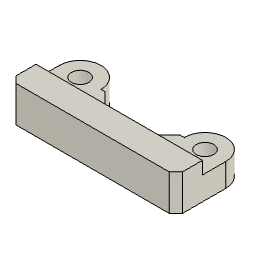
ADXL Nozzle Mount v8 (Autodesk Fusion 360 design; units mm, degrees)
Autodesk Fusion 360 part; units mm, degrees
note: some values were not read from the file. Set by a fixed rule: which sketch regions a step uses.
sketch "Sketch1" plane through (0, 0, 0) normal (0, 0, 1) x (1, 0, 0)
  circle A0 centre (-10.1925, 0) radius 2.5
  circle A1 centre (-25.1925, 0) radius 2.5
  circle A2 centre (-25.1925, 0) radius 1.6
  circle A3 centre (-10.1925, 0) radius 1.6
  line L0 (-27.6925, 0) -> (-7.6925, 0)
  line L1 (-7.6925, 0) -> (-7.6925, -6)
  line L2 (-7.6925, -6) -> (-27.6925, -6)
  line L3 (-27.6925, -6) -> (-27.6925, 0)
  line L4 (-27.6925, 0) -> (-22.6925, 0)
  line L5 (-20.6925, 0) -> (-14.6925, 0)
  line L6 (-14.6925, 0) -> (-14.6925, -2.5)
  line L7 (-14.6925, -2.5) -> (-20.6925, -2.5)
  line L8 (-20.6925, -2.5) -> (-20.6925, 0)
  line L9 (-27.6925, 0) -> (-2.5588, 0)
  line L10 (-7.6925, -2.8) -> (-27.6925, -2.8)
  line L11 (-27.6925, -2.8) -> (-27.6925, 0)
  circle A4 centre (-25.1925, 0) radius 1.05
  circle A5 centre (-10.1925, 0) radius 1.05
  dimension "d1" = 5
  dimension "d3" = 5
  dimension "d4" = 15
  dimension "d6" = 3.2
  dimension "d7" = 3.2
  dimension "d10" = 6
  dimension "d11" = 5
  dimension "d13" = 2.5
  dimension "d14" = 2.8
  dimension "d21" = 6
  dimension "d22" = 2.1
  dimension "d23" = 2.1
  constraint concentric A1 A2
  constraint concentric A0 A3
  constraint horizontal L0
  constraint coincident A1 L0.start
  constraint tangent A0 L1
  constraint horizontal L4
  constraint coincident L0 L5.start
  constraint midpoint L0 L5
  constraint coincident L1 L10.start
  constraint tangent A1 L3
  constraint perpendicular L1 L9
  constraint concentric A2 A4
  constraint concentric A0 A5
  measures "d1" diameter of A0
  measures "d3" diameter of A1
  measures "d4" distance of A0.centre A1.centre
  measures "d6" diameter of A2
  measures "d7" diameter of A3
  measures "d10" distance of L0.start L2.end
  measures "d11" distance of L0.start L4.end
  measures "d13" distance of L5.start L7.end
  measures "d14" distance of L0.start L10.end
  measures "d21" distance of L6 L8
  measures "d22" diameter of A4
  measures "d23" diameter of A5
extrude "Extrude1" add sketch "Sketch1" along normal blind 2.8 contours A0 A3 L0 L9 | A0 A1 L0 L1 L3 L6 L7 L8 L9 L10 L11 | A0 A3 L0 L9 | L1 L2 L3 L10 | A1 A2 L0 L4 L9 | A1 A2 L0 L4 L9
extrude "Extrude2" add sketch "Sketch1" along normal blind 4.32 contours L1 L2 L3 L10
chamfer "Chamfer1" distance 1.5 angle 45 2 edges at (-14.6925, 0, 1.4) (-20.6925, 0, 1.4)
chamfer "Chamfer2" distance 0.8 angle 45 2 edges at (-27.6925, -6, 2.16) (-7.6925, -6, 2.16)
extrude "Extrude3" add sketch "Sketch1" along normal up to surface (2.8 mm away) contours A3 L0 L9 A5 | A3 L0 L9 A5 | A2 L0 L4 L9 A4 | A2 L0 L4 L9 A4
equation "d17 = 2.8 mm + 1.52 mm"
